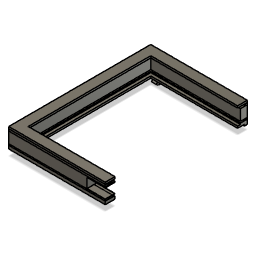
frame v12 (Autodesk Fusion 360 design; units mm, degrees)
Autodesk Fusion 360 part; units mm, degrees
note: some values were not read from the file. Chosen so that the rebuilt part matches the saved one: which bodies a step acts on; which face or edge a step refers to. Set by a fixed rule: which sketch regions a step uses.
sketch "Sketch1" plane through (0, 0, 0) normal (0, 1, 0) x (1, 0, 0)
  line L0 (178.39, 125.95) -> (-178.39, 125.95)
  line L1 (-178.39, 125.95) -> (-178.39, -125.95)
  line L2 (-178.39, -125.95) -> (178.39, -125.95)
  line L3 (178.39, -125.95) -> (178.39, 125.95)
  line L4 (178.39, 125.95) -> (-178.39, -125.95) construction
  line L5 (-178.39, 125.95) -> (178.39, -125.95) construction
  line L6 (198.39, 145.95) -> (-198.39, 145.95)
  line L7 (-198.39, 145.95) -> (-198.39, -145.95)
  line L8 (-198.39, -145.95) -> (198.39, -145.95)
  line L9 (198.39, -145.95) -> (198.39, 145.95)
  line L10 (198.39, 145.95) -> (-198.39, -145.95) construction
  line L11 (-198.39, 145.95) -> (198.39, -145.95) construction
  line L12 (-81.0361, 145.95) -> (-81.0361, 125.95) construction
  line L13 (-178.39, 44.0349) -> (-198.39, 44.0349) construction
  dimension "d1" = 356.78
  dimension "d2" = 251.9
  dimension "d3" = 20
  constraint horizontal L0
  constraint perpendicular L0 L1
  constraint parallel L0 L2
  constraint parallel L1 L3
  constraint coincident L4 origin
  constraint coincident L5 origin
  constraint horizontal L6
  constraint perpendicular L6 L7
  constraint parallel L6 L8
  constraint parallel L7 L9
  constraint coincident L10 origin
  constraint coincident L11 origin
  constraint coincident L6 L12.start
  constraint coincident L0 L12.end
  constraint perpendicular L0 L12
  constraint coincident L1 L13.start
  constraint coincident L7 L13.end
  constraint perpendicular L7 L13
  constraint equal L12 L13
  measures "d1" distance of L0.start L0.end
  measures "d2" distance of L0.start L2.end
  measures "d3" distance of L13.start L13.end
extrude "Extrude1" add sketch "Sketch1" along normal blind 40 makes body 1
sketch "Sketch9" plane through (0, 0, 0) normal (0, -1, 0) x (1, 0, 0)
  line L0 (178.39, 125.95) -> (178.39, -125.95)
  line L1 (178.39, -125.95) -> (-178.39, -125.95)
  line L2 (-178.39, -125.95) -> (-178.39, 125.95)
  line L3 (-178.39, 125.95) -> (178.39, 125.95)
  line L4 (198.39, -145.95) -> (198.39, 145.95)
  line L5 (198.39, 145.95) -> (-198.39, 145.95)
  line L6 (-198.39, 145.95) -> (-198.39, -145.95)
  line L7 (-198.39, -145.95) -> (198.39, -145.95)
  line L8 (-179.3845, -145.95) -> (180, -145.95)
  line L9 (180, -145.95) -> (180, -140)
  line L10 (180, -140) -> (-179.3845, -140)
  line L11 (-179.3845, -140) -> (-179.3845, -145.95)
  constraint horizontal L8
  constraint vertical L9
  constraint horizontal L10
  constraint vertical L11
  constraint coincident L7 L8.start
extrude "Extrude7" add sketch "Sketch9" along normal blind 3 contours L7 L8 L9 L10 L11 bodies 1
sketch "Sketch2" plane through (0, -3, 0) normal (0, -1, 0) x (1, 0, 0)
  line L0 (178.39, 125.95) -> (178.39, -125.95)
  line L1 (-178.39, -125.95) -> (-178.39, 125.95)
  line L2 (-178.39, 125.95) -> (178.39, 125.95)
  line L3 (198.39, -145.95) -> (198.39, 145.95)
  line L4 (198.39, 145.95) -> (-198.39, 145.95)
  line L5 (-198.39, 145.95) -> (-198.39, -145.95)
  line L6 (189.195, -145.95) -> (0, 0) construction
  line L7 (1298.9945, -150.8925) -> (475.6883, -150.8925)
  line L8 (-170, -145) -> (-180, -145)
  line L9 (-180, -145) -> (-180, -140)
  line L10 (-180, -140) -> (-170, -140)
  line L11 (-170, -140) -> (-170, -145)
  line L12 (198.39, -135.95) -> (-198.39, -135.95)
  line L13 (-178.39, -125.95) -> (178.39, -125.95)
  dimension "d33" = 10
  dimension "d34" = 10
  constraint coincident L6.end origin
  constraint horizontal L8
  constraint vertical L9
  constraint horizontal L10
  constraint vertical L11
  constraint coincident L3 L12.start
  constraint coincident L5 L12.end
  constraint perpendicular L5 L12
  measures "d33" distance of L12 L13
  measures "d34" distance of L8.start L8.end
revolve "Revolve1" add sketch "Sketch2" angle 145 about axis through (198.39, -3, -135.95) along (-1, 0, 0) contours L8 L9 L10 L11 bodies 1
sketch "Sketch3" plane through (0, 0, 145.95) normal (0, 0, 1) x (1, 0, 0)
  line L0 (-198.39, 0) -> (198.39, 0)
  line L1 (198.39, 0) -> (198.39, 40)
  line L2 (198.39, 40) -> (-198.39, 40)
  line L3 (-198.39, 40) -> (-198.39, 0)
  line L4 (-37.5, 30) -> (37.5, 30)
  line L5 (37.5, 30) -> (37.5, 10)
  line L6 (37.5, 10) -> (-37.5, 10)
  line L7 (-37.5, 10) -> (-37.5, 30)
  line L8 (0, 40) -> (0, 30) construction
  line L9 (0, 10) -> (0, 0) construction
  line L10 (-37.5, 18.9442) -> (-198.39, 18.9442) construction
  line L11 (37.5, 18.9442) -> (198.39, 18.9442) construction
  dimension "d10" = 20
  dimension "d11" = 75
  constraint horizontal L4
  constraint vertical L5
  constraint horizontal L6
  constraint vertical L7
  constraint midpoint L2 L8.start
  constraint coincident L4 L8.end
  constraint perpendicular L4 L8
  constraint coincident L6 L9.start
  constraint coincident L9.end origin
  constraint perpendicular L0 L9
  constraint equal L8 L9
  constraint coincident L7 L10.start
  constraint coincident L3 L10.end
  constraint perpendicular L3 L10
  constraint coincident L5 L11.start
  constraint coincident L1 L11.end
  constraint perpendicular L1 L11
  constraint equal L10 L11
  measures "d10" distance of L4.end L5.end
  measures "d11" distance of L4.start L4.end
extrude "Extrude2" cut sketch "Sketch3" against normal blind 30 contours L4 L5 L6 L7 bodies 1
sketch "Sketch4" plane through (0, 0, 125.95) normal (0, 0, -1) x (-1, 0, 0)
  line L0 (-37.5, 10) -> (-37.5, 30)
  line L1 (-37.5, 30) -> (37.5, 30)
  line L2 (37.5, 30) -> (37.5, 10)
  line L3 (37.5, 10) -> (-37.5, 10)
  line L4 (-178.39, 0) -> (178.39, 0)
  line L5 (178.39, 0) -> (178.39, 40)
  line L6 (178.39, 40) -> (-178.39, 40)
  line L7 (-178.39, 40) -> (-178.39, 0)
  line L8 (-38.5, 7.1767) -> (38.5, 7.1767)
  line L9 (38.5, 7.1767) -> (38.5, 5.4767)
  line L10 (38.5, 5.4767) -> (-38.5, 5.4767)
  line L11 (-38.5, 5.4767) -> (-38.5, 7.1767)
  line L12 (38.5, 5.4767) -> (178.39, 5.4767) construction
  line L13 (-38.5, 5.4767) -> (-178.39, 5.4767) construction
  dimension "d14" = 77
  dimension "d15" = 1.7
  constraint horizontal L8
  constraint vertical L9
  constraint horizontal L10
  constraint vertical L11
  constraint coincident L5 L12.end
  constraint perpendicular L5 L12
  constraint coincident L7 L13.end
  constraint perpendicular L7 L13
  constraint equal L12 L13
  measures "d14" distance of L9.end L10.end
  measures "d15" distance of L8.start L10.end
extrude "Extrude3" cut sketch "Sketch4" against normal blind 3 contours L8 L9 L10 L11 bodies 1
shell "Shell1" thickness 4 removed faces 4 at (59.4633, 13.3333, -125.95) at (-178.39, 13.3333, -41.9833) at (178.39, 13.3333, 41.9833) at (-131.76, 15.7256, 125.95) on bodies 1
sketch "Sketch7" plane through (0, 0, 125.95) normal (0, 0, -1) x (-1, 0, 0)
  line L0 (-37.5, 10) -> (-37.5, 30)
  line L1 (-37.5, 30) -> (37.5, 30)
  line L2 (37.5, 30) -> (37.5, 10)
  line L3 (37.5, 10) -> (-37.5, 10)
  line L4 (38.5, 7.1767) -> (38.5, 5.4767)
  line L5 (38.5, 5.4767) -> (-38.5, 5.4767)
  line L6 (-38.5, 5.4767) -> (-38.5, 7.1767)
  line L7 (-38.5, 7.1767) -> (38.5, 7.1767)
  line L8 (-178.39, 0) -> (178.39, 0)
  line L9 (-42.5, 35) -> (42.5, 35)
  line L10 (42.5, 35) -> (42.5, 32)
  line L11 (42.5, 32) -> (-42.5, 32)
  line L12 (-42.5, 32) -> (-42.5, 35)
  line L13 (-178.39, 4) -> (-178.39, 0)
  line L14 (178.39, 0) -> (178.39, 4)
  line L15 (-42.5, 4) -> (-178.39, 4)
  line L16 (178.39, 4) -> (42.5, 4)
  line L17 (42.5, 4) -> (42.5, 11.1767)
  line L18 (42.5, 11.1767) -> (41.5, 11.1767)
  line L19 (41.5, 11.1767) -> (41.5, 34)
  line L20 (41.5, 34) -> (-41.5, 34)
  line L21 (-41.5, 34) -> (-41.5, 11.1767)
  line L22 (-41.5, 11.1767) -> (-42.5, 11.1767)
  line L23 (-42.5, 11.1767) -> (-42.5, 4)
  dimension "d22" = 3
  dimension "d23" = 85
  constraint horizontal L9
  constraint vertical L10
  constraint horizontal L11
  constraint vertical L12
  measures "d22" distance of L9.start L11.end
  measures "d23" distance of L9.start L9.end
extrude "Extrude5" cut sketch "Sketch7" against normal blind 5 contours L11 L19 L20 L21 | L9 L10 L11 L12 L19 L20 L21 bodies 1
sketch "Sketch8" plane through (0, 0, 125.95) normal (0, 0, -1) x (-1, 0, 0)
  line L0 (41.5, 32) -> (-41.5, 32)
  line L1 (-178.39, 4) -> (-178.39, 0)
  line L2 (-178.39, 0) -> (178.39, 0)
  line L3 (178.39, 0) -> (178.39, 4)
  line L4 (38.5, 7.1767) -> (38.5, 5.4767)
  line L5 (38.5, 5.4767) -> (-38.5, 5.4767)
  line L6 (-38.5, 5.4767) -> (-38.5, 7.1767)
  line L7 (-38.5, 7.1767) -> (38.5, 7.1767)
  line L8 (-37.5, 10) -> (-37.5, 30)
  line L9 (-37.5, 30) -> (37.5, 30)
  line L10 (37.5, 30) -> (37.5, 10)
  line L11 (37.5, 10) -> (-37.5, 10)
  line L12 (-43.5, 9.3597) -> (43.5, 9.3597)
  line L13 (43.5, 9.3597) -> (43.5, 6.3597)
  line L14 (43.5, 6.3597) -> (-43.5, 6.3597)
  line L15 (-43.5, 6.3597) -> (-43.5, 9.3597)
  line L16 (-41.5, 32) -> (-41.5, 11.1767)
  line L17 (-41.5, 11.1767) -> (-42.5, 11.1767)
  line L18 (-42.5, 11.1767) -> (-42.5, 4)
  line L19 (-42.5, 4) -> (-178.39, 4)
  line L20 (178.39, 4) -> (42.5, 4)
  line L21 (42.5, 4) -> (42.5, 11.1767)
  line L22 (42.5, 11.1767) -> (41.5, 11.1767)
  line L23 (41.5, 11.1767) -> (41.5, 32)
  dimension "d26" = 3
  dimension "d27" = 87
  constraint horizontal L12
  constraint vertical L13
  constraint horizontal L14
  constraint vertical L15
  measures "d26" distance of L12.start L14.end
  measures "d27" distance of L12.start L12.end
extrude "Extrude6" cut sketch "Sketch8" against normal blind 5 contours L4 L6 L7 L12 L14 L18 L21 bodies 1
split "Split1" by plane through (0, 0, 0) normal (1, 0, 0) bodies 1 makes body 2 at (59.4633, 40, -135.3833)
move_body "Move1" bodies 2 to x (1, 0, 0) y (0, 1, 0) z (0, 0, 1) at (20, 0, 0)
split "Split2" by plane through (-41.5, 32, 125.95) normal (0, 1, 0) bodies 1 makes body 3 at (-59.4633, 40, -135.3833)
split "Split3" by plane through (20, 36, 0) normal (0, -1, 0) bodies 1 3 makes body 4 at (-13.8333, 32, 139.6167)
split "Split4" by plane through (-42.5, 6.3597, 125.95) normal (0, 1, 0) and through (42.5, 9.3597, 125.95) normal (0, -1, 0) bodies 1 makes body 5 at (-198.39, 16.9065, -48.65) makes body 6 at (-198.39, 7.3597, -48.65)
move_face "OffsetFaces1" offset 10 6 faces at (-58.4615, 5.5532, -141.95) (-194.39, 5.5732, -47.3167) (-144.1933, 5.4532, 141.95) (-64.7967, 24.4532, -141.95) (-143.4267, 24.4532, 141.95) (-194.39, 16.9065, -47.3167) on bodies 1 5
combine "Combine1" operation add target body 5 tool bodies 3 1 6 4 keep tools result as body 7 in component "Component"
component "Component" placed x (1, 0, 0) y (0, 1, 0) z (0, 0, 1) at (0, 0, 0)
hidden bodies 2
